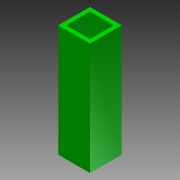
# Autodesk Inventor part: TabletMount-Mast-Lower
Saved by Autodesk Inventor 2012 (Build 160160000, 160)
## iProperties
Created: 2013-10-06
Part Number: TabletMount-Mast-Lower
Material: Default
Document SubType Name: Modeling
Designer: joe_000
Density: 1 g/cm^3
Author: joe_000
Autodesk Inventor part; units mm, degrees
ref_plane "YZ Plane" through (0, 0, 0) normal (1, 0, 0) x (0, 1, 0)
ref_plane "XZ Plane" through (0, 0, 0) normal (0, 1, 0) x (-1, 0, 0)
ref_plane "XY Plane" through (0, 0, 0) normal (0, 0, 1) x (1, 0, 0)
sketch "Sketch1" plane through (0, 0, 0) normal (0, 1, 0) x (-1, 0, 0)
  line L0 (0, 0) -> (19.05, 0)
  line L1 (19.05, 0) -> (19.05, -19.05)
  line L2 (19.05, -19.05) -> (0, -19.05)
  line L3 (0, -19.05) -> (0, 0)
  line L4 (-3.175, 3.175) -> (22.225, 3.175)
  line L5 (22.225, 3.175) -> (22.225, -22.225)
  line L6 (22.225, -22.225) -> (-3.175, -22.225)
  line L7 (-3.175, -22.225) -> (-3.175, 3.175)
  dimension "d0" = 19.05
  dimension "d1" = 19.05
  dimension "WallThickness" = 3.175
  dimension "d3" = 3.175
  dimension "d4" = 3.175
  dimension "d5" = 3.175
  constraints: 16 end point, 4 parallel, 2 horizontal, 2 perpendicular
  measures "d0" distance of L1.end L2.end
  measures "d1" distance of L0.end L1.end
  measures "WallThickness" distance between parallel lines of L1 L5
  measures "d3" distance between parallel lines of L0 L4
  measures "d4" distance between parallel lines of L7 L3
  measures "d5" distance between parallel lines of L6 L2
extrude "Extrusion1" add sketch "Sketch1" along normal blind 89.6112
equation "\"d0\" = MastWidth"
equation "\"d1\" = MastWidth"
equation "\"d3\" = WallThickness"
equation "\"d4\" = WallThickness"
equation "\"d5\" = WallThickness"
equation "\"d6\" = ServoMountLength"
equation "\"MastWidth\" = 19.05"
equation "\"ServoMountLength\" = 89.6112"
body "Solid1"
